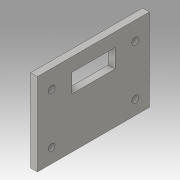
# Autodesk Inventor part: SwitchBracket
Saved by Autodesk Inventor 2016 (Build 200138000, 138)
## iProperties
Created: 2016-11-05
Part Number: SwitchBracket
Material: Generic
Document SubType Name: Modeling
Designer: Delta
Density: 1 g/cm^3
Appearance: Default
Author: Delta
Autodesk Inventor part; units mm, degrees
ref_plane "YZ Plane" through (0, 0, 0) normal (1, 0, 0) x (0, 1, 0)
ref_plane "XZ Plane" through (0, 0, 0) normal (0, 1, 0) x (-1, 0, 0)
ref_plane "XY Plane" through (0, 0, 0) normal (0, 0, 1) x (1, 0, 0)
sketch "Sketch1" plane through (0, 0, 0) normal (1, 0, 0) x (0, 1, 0)
  line L0 (0, 0) -> (58.0898, 0)
  line L1 (58.0898, 0) -> (58.0898, -78.7908)
  line L2 (58.0898, -78.7908) -> (0, -78.7908)
  line L3 (0, -78.7908) -> (0, 0)
  dimension "d0" = 78.7908
  dimension "d1" = 58.0898
  constraints: 8 end point, 2 parallel, 1 horizontal, 1 perpendicular
  measures "d0" distance of L0.end L1.end
  measures "d1" distance of L0.start L0.end
extrude "Extrusion1" add sketch "Sketch1" along normal blind 4.7752
sketch "Sketch2" plane through (4.7752, 0, 0) normal (1, 0, 0) x (0, 0, -1)
  line L0 (0, 58.0898) -> (0, 0) projected
  line L1 (78.7908, 58.0898) -> (0, 58.0898) projected
  line L2 (0, 0) -> (78.7908, 0) projected
  line L3 (78.7908, 0) -> (78.7908, 58.0898) projected
  point P0 (10, 45.3898)
  point P1 (68.7908, 45.3898)
  point P2 (10, 10)
  point P3 (68.7908, 10)
  dimension "d4" = 10
  dimension "d6" = 10
  dimension "d7" = 10
  dimension "d9" = 10
  dimension "d10" = 12.7
  dimension "d12" = 12.7
  dimension "d16" = 10
  dimension "d17" = 10
  measures "d4" distance from line of L0 point (10, 45.39)
  measures "d6" distance from line of L2 point (10, 10)
  measures "d7" distance from line of L2 point (68.791, 10)
  measures "d9" distance from line of L3 point (68.791, 45.39)
  measures "d10" distance from line of point (10, 45.39) L1
  measures "d12" distance from line of L1 point (68.791, 45.39)
  measures "d16" distance from line of L0 point (10, 10)
  measures "d17" distance from line of L3 point (68.791, 10)
hole "Hole1" at (4.7752, 45.3898, -10) at (4.7752, 45.3898, -68.7908) at (4.7752, 10, -10) at (4.7752, 10, -68.7908) direction (-1, 0, 0) diameter 4.7752 end through all
sketch "Sketch3" plane through (4.7752, 0, 0) normal (1, 0, 0) x (0, 0, -1)
  line L0 (24.1554, 35.4838) -> (54.6354, 35.4838)
  line L1 (54.6354, 35.4838) -> (54.6354, 48.5648)
  line L2 (54.6354, 48.5648) -> (24.1554, 48.5648)
  line L3 (24.1554, 48.5648) -> (24.1554, 35.4838)
  line L4 (0, 58.0898) -> (0, 0) projected
  line L5 (78.7908, 58.0898) -> (0, 58.0898) projected
  dimension "d25" = 13.081
  dimension "d26" = 30.48
  dimension "d28" = 78.7908
  dimension "d29" = 24.1554
  dimension "d30" = 58.0898
  dimension "d31" = 9.525
  constraints: 8 end point, 2 parallel, 1 horizontal, 1 perpendicular
  measures "d25" distance of L2.end L0.start
  measures "d26" distance of L1.end L2.end
  measures "d28" distance of L5.start L4.start
  measures "d29" distance between parallel lines of L4 L3
  measures "d30" distance of L4.start L4.end
  measures "d31" distance between parallel lines of L5 L2
extrude "Extrusion2" cut sketch "Sketch3" against normal through all
equation "\"d29\" = -0.5 * d26 + 0.5 * d28"
body "Solid1"
